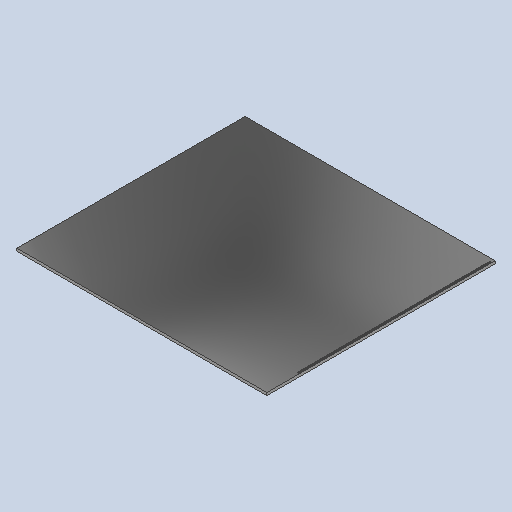
# Autodesk Inventor part: ETROC2
Saved by Autodesk Inventor 2022 (Build 260153000, 153)
## iProperties
Created: 2022-02-01
Part Number: ETROC2
Material: Silicon Nitride
Document SubType Name: Modeling
Designer: Caleb
Density: 3.18 g/cm^3
Appearance: Chrome - Polished Black
Author: Caleb
Autodesk Inventor part; units mm, degrees
ref_plane "YZ Plane" through (0, 0, 0) normal (1, 0, 0) x (0, 1, 0)
ref_plane "XZ Plane" through (0, 0, 0) normal (0, 1, 0) x (-1, 0, 0)
ref_plane "XY Plane" through (0, 0, 0) normal (0, 0, 1) x (1, 0, 0)
sketch "Sketch1" plane through (0, 0, 0) normal (0, 1, 0) x (-1, 0, 0)
  point P0 (0, 0)
sketch "Sketch2" plane through (0, 0, 0) normal (0, 1, 0) x (-1, 0, 0)
  line L0 (-11.5, 10.5) -> (11.5, 10.5)
  line L1 (11.5, 10.5) -> (11.5, -10.5)
  line L2 (11.5, -10.5) -> (-11.5, -10.5)
  line L3 (-11.5, -10.5) -> (-11.5, 10.5)
  line L4 (-11.5, 10.5) -> (11.5, -10.5) construction
  line L5 (11.5, 10.5) -> (-11.5, -10.5) construction
  point P0 (0, 0)
  dimension "d0" = 21
  dimension "d1" = 23
  constraints: 12 end point, 2 midpoint, 2 parallel, 1 horizontal, 1 perpendicular
  measures "d0" distance of L0.end L1.end
  measures "d1" distance of L0.start L0.end
extrude "Extrusion1" add sketch "Sketch2" along normal blind 0.25
sketch "Sketch3" plane through (0, 0.25, 0) normal (0, 1, 0) x (1, 0, 0)
  line L0 (11.5, -10.5) -> (11.5, 10.5) projected
  line L1 (-11.5, -10.5) -> (11.5, -10.5) projected
  line L2 (11.45, -7.5) -> (11.3, -7.5)
  line L3 (11.3, -7.5) -> (11.3, -7.42)
  line L4 (11.3, -7.42) -> (11.45, -7.42)
  line L5 (11.45, -7.42) -> (11.45, -7.5)
  line L6 (11.45, -7.5) -> (11.3, -7.42) construction
  line L7 (11.3, -7.5) -> (11.45, -7.42) construction
  line L8 (11.45, -7.375) -> (11.3, -7.375)
  line L9 (11.3, -7.375) -> (11.3, -7.295)
  line L10 (11.3, -7.295) -> (11.45, -7.295)
  line L11 (11.45, -7.295) -> (11.45, -7.375)
  line L12 (11.45, -7.375) -> (11.3, -7.295) construction
  line L13 (11.3, -7.375) -> (11.45, -7.295) construction
  line L14 (11.45, -7.25) -> (11.3, -7.25)
  line L15 (11.3, -7.25) -> (11.3, -7.17)
  line L16 (11.3, -7.17) -> (11.45, -7.17)
  line L17 (11.45, -7.17) -> (11.45, -7.25)
  line L18 (11.45, -7.25) -> (11.3, -7.17) construction
  line L19 (11.3, -7.25) -> (11.45, -7.17) construction
  line L20 (11.45, -7.125) -> (11.3, -7.125)
  line L21 (11.3, -7.125) -> (11.3, -7.045)
  line L22 (11.3, -7.045) -> (11.45, -7.045)
  line L23 (11.45, -7.045) -> (11.45, -7.125)
  line L24 (11.45, -7.125) -> (11.3, -7.045) construction
  line L25 (11.3, -7.125) -> (11.45, -7.045) construction
  line L26 (11.45, -7) -> (11.3, -7)
  line L27 (11.3, -7) -> (11.3, -6.92)
  line L28 (11.3, -6.92) -> (11.45, -6.92)
  line L29 (11.45, -6.92) -> (11.45, -7)
  line L30 (11.45, -7) -> (11.3, -6.92) construction
  line L31 (11.3, -7) -> (11.45, -6.92) construction
  line L32 (11.45, -6.875) -> (11.3, -6.875)
  line L33 (11.3, -6.875) -> (11.3, -6.795)
  line L34 (11.3, -6.795) -> (11.45, -6.795)
  line L35 (11.45, -6.795) -> (11.45, -6.875)
  line L36 (11.45, -6.875) -> (11.3, -6.795) construction
  line L37 (11.3, -6.875) -> (11.45, -6.795) construction
  line L38 (11.45, -6.75) -> (11.3, -6.75)
  line L39 (11.3, -6.75) -> (11.3, -6.67)
  line L40 (11.3, -6.67) -> (11.45, -6.67)
  line L41 (11.45, -6.67) -> (11.45, -6.75)
  line L42 (11.45, -6.75) -> (11.3, -6.67) construction
  line L43 (11.3, -6.75) -> (11.45, -6.67) construction
  line L44 (11.45, -6.625) -> (11.3, -6.625)
  line L45 (11.3, -6.625) -> (11.3, -6.545)
  line L46 (11.3, -6.545) -> (11.45, -6.545)
  line L47 (11.45, -6.545) -> (11.45, -6.625)
  line L48 (11.45, -6.625) -> (11.3, -6.545) construction
  line L49 (11.3, -6.625) -> (11.45, -6.545) construction
  line L50 (11.45, -6.5) -> (11.3, -6.5)
  line L51 (11.3, -6.5) -> (11.3, -6.42)
  line L52 (11.3, -6.42) -> (11.45, -6.42)
  line L53 (11.45, -6.42) -> (11.45, -6.5)
  line L54 (11.45, -6.5) -> (11.3, -6.42) construction
  line L55 (11.3, -6.5) -> (11.45, -6.42) construction
  line L56 (11.45, -6.375) -> (11.3, -6.375)
  line L57 (11.3, -6.375) -> (11.3, -6.295)
  line L58 (11.3, -6.295) -> (11.45, -6.295)
  line L59 (11.45, -6.295) -> (11.45, -6.375)
  line L60 (11.45, -6.375) -> (11.3, -6.295) construction
  line L61 (11.3, -6.375) -> (11.45, -6.295) construction
  line L62 (11.45, -6.25) -> (11.3, -6.25)
  line L63 (11.3, -6.25) -> (11.3, -6.17)
  line L64 (11.3, -6.17) -> (11.45, -6.17)
  line L65 (11.45, -6.17) -> (11.45, -6.25)
  line L66 (11.45, -6.25) -> (11.3, -6.17) construction
  line L67 (11.3, -6.25) -> (11.45, -6.17) construction
  line L68 (11.45, -6.125) -> (11.3, -6.125)
  line L69 (11.3, -6.125) -> (11.3, -6.045)
  line L70 (11.3, -6.045) -> (11.45, -6.045)
  line L71 (11.45, -6.045) -> (11.45, -6.125)
  line L72 (11.45, -6.125) -> (11.3, -6.045) construction
  line L73 (11.3, -6.125) -> (11.45, -6.045) construction
  line L74 (11.45, -6) -> (11.3, -6)
  line L75 (11.3, -6) -> (11.3, -5.92)
  line L76 (11.3, -5.92) -> (11.45, -5.92)
  line L77 (11.45, -5.92) -> (11.45, -6)
  line L78 (11.45, -6) -> (11.3, -5.92) construction
  line L79 (11.3, -6) -> (11.45, -5.92) construction
  line L80 (11.45, -5.875) -> (11.3, -5.875)
  line L81 (11.3, -5.875) -> (11.3, -5.795)
  line L82 (11.3, -5.795) -> (11.45, -5.795)
  line L83 (11.45, -5.795) -> (11.45, -5.875)
  line L84 (11.45, -5.875) -> (11.3, -5.795) construction
  line L85 (11.3, -5.875) -> (11.45, -5.795) construction
  line L86 (11.45, -5.75) -> (11.3, -5.75)
  line L87 (11.3, -5.75) -> (11.3, -5.67)
  line L88 (11.3, -5.67) -> (11.45, -5.67)
  line L89 (11.45, -5.67) -> (11.45, -5.75)
  line L90 (11.45, -5.75) -> (11.3, -5.67) construction
  line L91 (11.3, -5.75) -> (11.45, -5.67) construction
  line L92 (11.45, -5.625) -> (11.3, -5.625)
  line L93 (11.3, -5.625) -> (11.3, -5.545)
  line L94 (11.3, -5.545) -> (11.45, -5.545)
  line L95 (11.45, -5.545) -> (11.45, -5.625)
  line L96 (11.45, -5.625) -> (11.3, -5.545) construction
  line L97 (11.3, -5.625) -> (11.45, -5.545) construction
  line L98 (11.45, -5.5) -> (11.3, -5.5)
  line L99 (11.3, -5.5) -> (11.3, -5.42)
  line L100 (11.3, -5.42) -> (11.45, -5.42)
  line L101 (11.45, -5.42) -> (11.45, -5.5)
  line L102 (11.45, -5.5) -> (11.3, -5.42) construction
  line L103 (11.3, -5.5) -> (11.45, -5.42) construction
  line L104 (11.45, -5.375) -> (11.3, -5.375)
  line L105 (11.3, -5.375) -> (11.3, -5.295)
  line L106 (11.3, -5.295) -> (11.45, -5.295)
  line L107 (11.45, -5.295) -> (11.45, -5.375)
  line L108 (11.45, -5.375) -> (11.3, -5.295) construction
  line L109 (11.3, -5.375) -> (11.45, -5.295) construction
  line L110 (11.45, -5.25) -> (11.3, -5.25)
  line L111 (11.3, -5.25) -> (11.3, -5.17)
  line L112 (11.3, -5.17) -> (11.45, -5.17)
  line L113 (11.45, -5.17) -> (11.45, -5.25)
  line L114 (11.45, -5.25) -> (11.3, -5.17) construction
  line L115 (11.3, -5.25) -> (11.45, -5.17) construction
  line L116 (11.45, -5.125) -> (11.3, -5.125)
  line L117 (11.3, -5.125) -> (11.3, -5.045)
  line L118 (11.3, -5.045) -> (11.45, -5.045)
  line L119 (11.45, -5.045) -> (11.45, -5.125)
  line L120 (11.45, -5.125) -> (11.3, -5.045) construction
  line L121 (11.3, -5.125) -> (11.45, -5.045) construction
  line L122 (11.45, -5) -> (11.3, -5)
  line L123 (11.3, -5) -> (11.3, -4.92)
  line L124 (11.3, -4.92) -> (11.45, -4.92)
  line L125 (11.45, -4.92) -> (11.45, -5)
  line L126 (11.45, -5) -> (11.3, -4.92) construction
  line L127 (11.3, -5) -> (11.45, -4.92) construction
  line L128 (11.45, -4.875) -> (11.3, -4.875)
  line L129 (11.3, -4.875) -> (11.3, -4.795)
  line L130 (11.3, -4.795) -> (11.45, -4.795)
  line L131 (11.45, -4.795) -> (11.45, -4.875)
  line L132 (11.45, -4.875) -> (11.3, -4.795) construction
  line L133 (11.3, -4.875) -> (11.45, -4.795) construction
  line L134 (11.45, -4.75) -> (11.3, -4.75)
  line L135 (11.3, -4.75) -> (11.3, -4.67)
  line L136 (11.3, -4.67) -> (11.45, -4.67)
  line L137 (11.45, -4.67) -> (11.45, -4.75)
  line L138 (11.45, -4.75) -> (11.3, -4.67) construction
  line L139 (11.3, -4.75) -> (11.45, -4.67) construction
  line L140 (11.45, -4.625) -> (11.3, -4.625)
  line L141 (11.3, -4.625) -> (11.3, -4.545)
  line L142 (11.3, -4.545) -> (11.45, -4.545)
  line L143 (11.45, -4.545) -> (11.45, -4.625)
  line L144 (11.45, -4.625) -> (11.3, -4.545) construction
  line L145 (11.3, -4.625) -> (11.45, -4.545) construction
  line L146 (11.45, -4.5) -> (11.3, -4.5)
  line L147 (11.3, -4.5) -> (11.3, -4.42)
  line L148 (11.3, -4.42) -> (11.45, -4.42)
  line L149 (11.45, -4.42) -> (11.45, -4.5)
  line L150 (11.45, -4.5) -> (11.3, -4.42) construction
  line L151 (11.3, -4.5) -> (11.45, -4.42) construction
  line L152 (11.45, -4.375) -> (11.3, -4.375)
  line L153 (11.3, -4.375) -> (11.3, -4.295)
  line L154 (11.3, -4.295) -> (11.45, -4.295)
  line L155 (11.45, -4.295) -> (11.45, -4.375)
  line L156 (11.45, -4.375) -> (11.3, -4.295) construction
  line L157 (11.3, -4.375) -> (11.45, -4.295) construction
  line L158 (11.45, -4.25) -> (11.3, -4.25)
  line L159 (11.3, -4.25) -> (11.3, -4.17)
  line L160 (11.3, -4.17) -> (11.45, -4.17)
  line L161 (11.45, -4.17) -> (11.45, -4.25)
  line L162 (11.45, -4.25) -> (11.3, -4.17) construction
  line L163 (11.3, -4.25) -> (11.45, -4.17) construction
  line L164 (11.45, -4.125) -> (11.3, -4.125)
  line L165 (11.3, -4.125) -> (11.3, -4.045)
  line L166 (11.3, -4.045) -> (11.45, -4.045)
  line L167 (11.45, -4.045) -> (11.45, -4.125)
  line L168 (11.45, -4.125) -> (11.3, -4.045) construction
  line L169 (11.3, -4.125) -> (11.45, -4.045) construction
  line L170 (11.45, -4) -> (11.3, -4)
  line L171 (11.3, -4) -> (11.3, -3.92)
  line L172 (11.3, -3.92) -> (11.45, -3.92)
  line L173 (11.45, -3.92) -> (11.45, -4)
  line L174 (11.45, -4) -> (11.3, -3.92) construction
  line L175 (11.3, -4) -> (11.45, -3.92) construction
  line L176 (11.45, -3.875) -> (11.3, -3.875)
  line L177 (11.3, -3.875) -> (11.3, -3.795)
  line L178 (11.3, -3.795) -> (11.45, -3.795)
  line L179 (11.45, -3.795) -> (11.45, -3.875)
  line L180 (11.45, -3.875) -> (11.3, -3.795) construction
  line L181 (11.3, -3.875) -> (11.45, -3.795) construction
  line L182 (11.45, -3.75) -> (11.3, -3.75)
  line L183 (11.3, -3.75) -> (11.3, -3.67)
  line L184 (11.3, -3.67) -> (11.45, -3.67)
  line L185 (11.45, -3.67) -> (11.45, -3.75)
  line L186 (11.45, -3.75) -> (11.3, -3.67) construction
  line L187 (11.3, -3.75) -> (11.45, -3.67) construction
  line L188 (11.45, -3.625) -> (11.3, -3.625)
  line L189 (11.3, -3.625) -> (11.3, -3.545)
  line L190 (11.3, -3.545) -> (11.45, -3.545)
  line L191 (11.45, -3.545) -> (11.45, -3.625)
  line L192 (11.45, -3.625) -> (11.3, -3.545) construction
  line L193 (11.3, -3.625) -> (11.45, -3.545) construction
  line L194 (11.45, -3.5) -> (11.3, -3.5)
  line L195 (11.3, -3.5) -> (11.3, -3.42)
  line L196 (11.3, -3.42) -> (11.45, -3.42)
  line L197 (11.45, -3.42) -> (11.45, -3.5)
  line L198 (11.45, -3.5) -> (11.3, -3.42) construction
  line L199 (11.3, -3.5) -> (11.45, -3.42) construction
  line L200 (11.45, -3.375) -> (11.3, -3.375)
  line L201 (11.3, -3.375) -> (11.3, -3.295)
  line L202 (11.3, -3.295) -> (11.45, -3.295)
  line L203 (11.45, -3.295) -> (11.45, -3.375)
  line L204 (11.45, -3.375) -> (11.3, -3.295) construction
  line L205 (11.3, -3.375) -> (11.45, -3.295) construction
  line L206 (11.45, -3.25) -> (11.3, -3.25)
  line L207 (11.3, -3.25) -> (11.3, -3.17)
  line L208 (11.3, -3.17) -> (11.45, -3.17)
  line L209 (11.45, -3.17) -> (11.45, -3.25)
  line L210 (11.45, -3.25) -> (11.3, -3.17) construction
  line L211 (11.3, -3.25) -> (11.45, -3.17) construction
  line L212 (11.45, -3.125) -> (11.3, -3.125)
  line L213 (11.3, -3.125) -> (11.3, -3.045)
  line L214 (11.3, -3.045) -> (11.45, -3.045)
  line L215 (11.45, -3.045) -> (11.45, -3.125)
  line L216 (11.45, -3.125) -> (11.3, -3.045) construction
  line L217 (11.3, -3.125) -> (11.45, -3.045) construction
  line L218 (11.45, -3) -> (11.3, -3)
  line L219 (11.3, -3) -> (11.3, -2.92)
  line L220 (11.3, -2.92) -> (11.45, -2.92)
  line L221 (11.45, -2.92) -> (11.45, -3)
  line L222 (11.45, -3) -> (11.3, -2.92) construction
  line L223 (11.3, -3) -> (11.45, -2.92) construction
  line L224 (11.45, -2.875) -> (11.3, -2.875)
  line L225 (11.3, -2.875) -> (11.3, -2.795)
  line L226 (11.3, -2.795) -> (11.45, -2.795)
  line L227 (11.45, -2.795) -> (11.45, -2.875)
  line L228 (11.45, -2.875) -> (11.3, -2.795) construction
  line L229 (11.3, -2.875) -> (11.45, -2.795) construction
  line L230 (11.45, -2.75) -> (11.3, -2.75)
  line L231 (11.3, -2.75) -> (11.3, -2.67)
  line L232 (11.3, -2.67) -> (11.45, -2.67)
  line L233 (11.45, -2.67) -> (11.45, -2.75)
  line L234 (11.45, -2.75) -> (11.3, -2.67) construction
  line L235 (11.3, -2.75) -> (11.45, -2.67) construction
  line L236 (11.45, -2.625) -> (11.3, -2.625)
  line L237 (11.3, -2.625) -> (11.3, -2.545)
  line L238 (11.3, -2.545) -> (11.45, -2.545)
  line L239 (11.45, -2.545) -> (11.45, -2.625)
  line L240 (11.45, -2.625) -> (11.3, -2.545) construction
  line L241 (11.3, -2.625) -> (11.45, -2.545) construction
  line L242 (11.45, -2.5) -> (11.3, -2.5)
  line L243 (11.3, -2.5) -> (11.3, -2.42)
  line L244 (11.3, -2.42) -> (11.45, -2.42)
  line L245 (11.45, -2.42) -> (11.45, -2.5)
  line L246 (11.45, -2.5) -> (11.3, -2.42) construction
  line L247 (11.3, -2.5) -> (11.45, -2.42) construction
  line L248 (11.45, -2.375) -> (11.3, -2.375)
  line L249 (11.3, -2.375) -> (11.3, -2.295)
  line L250 (11.3, -2.295) -> (11.45, -2.295)
  line L251 (11.45, -2.295) -> (11.45, -2.375)
  line L252 (11.45, -2.375) -> (11.3, -2.295) construction
  line L253 (11.3, -2.375) -> (11.45, -2.295) construction
  line L254 (11.45, -2.25) -> (11.3, -2.25)
  line L255 (11.3, -2.25) -> (11.3, -2.17)
  line L256 (11.3, -2.17) -> (11.45, -2.17)
  line L257 (11.45, -2.17) -> (11.45, -2.25)
  line L258 (11.45, -2.25) -> (11.3, -2.17) construction
  line L259 (11.3, -2.25) -> (11.45, -2.17) construction
  line L260 (11.45, -2.125) -> (11.3, -2.125)
  line L261 (11.3, -2.125) -> (11.3, -2.045)
  line L262 (11.3, -2.045) -> (11.45, -2.045)
  line L263 (11.45, -2.045) -> (11.45, -2.125)
  line L264 (11.45, -2.125) -> (11.3, -2.045) construction
  line L265 (11.3, -2.125) -> (11.45, -2.045) construction
  line L266 (11.45, -2) -> (11.3, -2)
  line L267 (11.3, -2) -> (11.3, -1.92)
  line L268 (11.3, -1.92) -> (11.45, -1.92)
  line L269 (11.45, -1.92) -> (11.45, -2)
  line L270 (11.45, -2) -> (11.3, -1.92) construction
  line L271 (11.3, -2) -> (11.45, -1.92) construction
  line L272 (11.45, -1.875) -> (11.3, -1.875)
  line L273 (11.3, -1.875) -> (11.3, -1.795)
  line L274 (11.3, -1.795) -> (11.45, -1.795)
  line L275 (11.45, -1.795) -> (11.45, -1.875)
  line L276 (11.45, -1.875) -> (11.3, -1.795) construction
  line L277 (11.3, -1.875) -> (11.45, -1.795) construction
  line L278 (11.45, -1.75) -> (11.3, -1.75)
  line L279 (11.3, -1.75) -> (11.3, -1.67)
  line L280 (11.3, -1.67) -> (11.45, -1.67)
  line L281 (11.45, -1.67) -> (11.45, -1.75)
  line L282 (11.45, -1.75) -> (11.3, -1.67) construction
  line L283 (11.3, -1.75) -> (11.45, -1.67) construction
  line L284 (11.45, -1.625) -> (11.3, -1.625)
  line L285 (11.3, -1.625) -> (11.3, -1.545)
  line L286 (11.3, -1.545) -> (11.45, -1.545)
  line L287 (11.45, -1.545) -> (11.45, -1.625)
  line L288 (11.45, -1.625) -> (11.3, -1.545) construction
  line L289 (11.3, -1.625) -> (11.45, -1.545) construction
  line L290 (11.45, -1.5) -> (11.3, -1.5)
  line L291 (11.3, -1.5) -> (11.3, -1.42)
  line L292 (11.3, -1.42) -> (11.45, -1.42)
  line L293 (11.45, -1.42) -> (11.45, -1.5)
  line L294 (11.45, -1.5) -> (11.3, -1.42) construction
  line L295 (11.3, -1.5) -> (11.45, -1.42) construction
  line L296 (11.45, -1.375) -> (11.3, -1.375)
  line L297 (11.3, -1.375) -> (11.3, -1.295)
  line L298 (11.3, -1.295) -> (11.45, -1.295)
  line L299 (11.45, -1.295) -> (11.45, -1.375)
  line L300 (11.45, -1.375) -> (11.3, -1.295) construction
  line L301 (11.3, -1.375) -> (11.45, -1.295) construction
  line L302 (11.45, -1.25) -> (11.3, -1.25)
  line L303 (11.3, -1.25) -> (11.3, -1.17)
  line L304 (11.3, -1.17) -> (11.45, -1.17)
  line L305 (11.45, -1.17) -> (11.45, -1.25)
  line L306 (11.45, -1.25) -> (11.3, -1.17) construction
  line L307 (11.3, -1.25) -> (11.45, -1.17) construction
  line L308 (11.45, -1.125) -> (11.3, -1.125)
  line L309 (11.3, -1.125) -> (11.3, -1.045)
  line L310 (11.3, -1.045) -> (11.45, -1.045)
  line L311 (11.45, -1.045) -> (11.45, -1.125)
  line L312 (11.45, -1.125) -> (11.3, -1.045) construction
  line L313 (11.3, -1.125) -> (11.45, -1.045) construction
  line L314 (11.45, -1) -> (11.3, -1)
  line L315 (11.3, -1) -> (11.3, -0.92)
  line L316 (11.3, -0.92) -> (11.45, -0.92)
  line L317 (11.45, -0.92) -> (11.45, -1)
  line L318 (11.45, -1) -> (11.3, -0.92) construction
  line L319 (11.3, -1) -> (11.45, -0.92) construction
  line L320 (11.45, -0.875) -> (11.3, -0.875)
  line L321 (11.3, -0.875) -> (11.3, -0.795)
  line L322 (11.3, -0.795) -> (11.45, -0.795)
  line L323 (11.45, -0.795) -> (11.45, -0.875)
  line L324 (11.45, -0.875) -> (11.3, -0.795) construction
  line L325 (11.3, -0.875) -> (11.45, -0.795) construction
  line L326 (11.45, -0.75) -> (11.3, -0.75)
  line L327 (11.3, -0.75) -> (11.3, -0.67)
  line L328 (11.3, -0.67) -> (11.45, -0.67)
  line L329 (11.45, -0.67) -> (11.45, -0.75)
  line L330 (11.45, -0.75) -> (11.3, -0.67) construction
  line L331 (11.3, -0.75) -> (11.45, -0.67) construction
  line L332 (11.45, -0.625) -> (11.3, -0.625)
  line L333 (11.3, -0.625) -> (11.3, -0.545)
  line L334 (11.3, -0.545) -> (11.45, -0.545)
  line L335 (11.45, -0.545) -> (11.45, -0.625)
  line L336 (11.45, -0.625) -> (11.3, -0.545) construction
  line L337 (11.3, -0.625) -> (11.45, -0.545) construction
  line L338 (11.45, -0.5) -> (11.3, -0.5)
  line L339 (11.3, -0.5) -> (11.3, -0.42)
  line L340 (11.3, -0.42) -> (11.45, -0.42)
  line L341 (11.45, -0.42) -> (11.45, -0.5)
  line L342 (11.45, -0.5) -> (11.3, -0.42) construction
  line L343 (11.3, -0.5) -> (11.45, -0.42) construction
  line L344 (11.45, -0.375) -> (11.3, -0.375)
  line L345 (11.3, -0.375) -> (11.3, -0.295)
  line L346 (11.3, -0.295) -> (11.45, -0.295)
  line L347 (11.45, -0.295) -> (11.45, -0.375)
  line L348 (11.45, -0.375) -> (11.3, -0.295) construction
  line L349 (11.3, -0.375) -> (11.45, -0.295) construction
  line L350 (11.45, -0.25) -> (11.3, -0.25)
  line L351 (11.3, -0.25) -> (11.3, -0.17)
  line L352 (11.3, -0.17) -> (11.45, -0.17)
  line L353 (11.45, -0.17) -> (11.45, -0.25)
  line L354 (11.45, -0.25) -> (11.3, -0.17) construction
  line L355 (11.3, -0.25) -> (11.45, -0.17) construction
  line L356 (11.45, -0.125) -> (11.3, -0.125)
  line L357 (11.3, -0.125) -> (11.3, -0.045)
  line L358 (11.3, -0.045) -> (11.45, -0.045)
  line L359 (11.45, -0.045) -> (11.45, -0.125)
  line L360 (11.45, -0.125) -> (11.3, -0.045) construction
  line L361 (11.3, -0.125) -> (11.45, -0.045) construction
  line L362 (11.45, 0) -> (11.3, 0)
  line L363 (11.3, 0) -> (11.3, 0.08)
  line L364 (11.3, 0.08) -> (11.45, 0.08)
  line L365 (11.45, 0.08) -> (11.45, 0)
  line L366 (11.45, 0) -> (11.3, 0.08) construction
  line L367 (11.3, 0) -> (11.45, 0.08) construction
  line L368 (11.45, 0.125) -> (11.3, 0.125)
  line L369 (11.3, 0.125) -> (11.3, 0.205)
  line L370 (11.3, 0.205) -> (11.45, 0.205)
  line L371 (11.45, 0.205) -> (11.45, 0.125)
  line L372 (11.45, 0.125) -> (11.3, 0.205) construction
  line L373 (11.3, 0.125) -> (11.45, 0.205) construction
  line L374 (11.45, 0.25) -> (11.3, 0.25)
  line L375 (11.3, 0.25) -> (11.3, 0.33)
  line L376 (11.3, 0.33) -> (11.45, 0.33)
  line L377 (11.45, 0.33) -> (11.45, 0.25)
  line L378 (11.45, 0.25) -> (11.3, 0.33) construction
  line L379 (11.3, 0.25) -> (11.45, 0.33) construction
  line L380 (11.45, 0.375) -> (11.3, 0.375)
  line L381 (11.3, 0.375) -> (11.3, 0.455)
  line L382 (11.3, 0.455) -> (11.45, 0.455)
  line L383 (11.45, 0.455) -> (11.45, 0.375)
  line L384 (11.45, 0.375) -> (11.3, 0.455) construction
  line L385 (11.3, 0.375) -> (11.45, 0.455) construction
  line L386 (11.45, 0.5) -> (11.3, 0.5)
  line L387 (11.3, 0.5) -> (11.3, 0.58)
  line L388 (11.3, 0.58) -> (11.45, 0.58)
  line L389 (11.45, 0.58) -> (11.45, 0.5)
  line L390 (11.45, 0.5) -> (11.3, 0.58) construction
  line L391 (11.3, 0.5) -> (11.45, 0.58) construction
  line L392 (11.45, 0.625) -> (11.3, 0.625)
  line L393 (11.3, 0.625) -> (11.3, 0.705)
  line L394 (11.3, 0.705) -> (11.45, 0.705)
  line L395 (11.45, 0.705) -> (11.45, 0.625)
  line L396 (11.45, 0.625) -> (11.3, 0.705) construction
  line L397 (11.3, 0.625) -> (11.45, 0.705) construction
  line L398 (11.45, 0.75) -> (11.3, 0.75)
  line L399 (11.3, 0.75) -> (11.3, 0.83)
  line L400 (11.3, 0.83) -> (11.45, 0.83)
  line L401 (11.45, 0.83) -> (11.45, 0.75)
  line L402 (11.45, 0.75) -> (11.3, 0.83) construction
  line L403 (11.3, 0.75) -> (11.45, 0.83) construction
  line L404 (11.45, 0.875) -> (11.3, 0.875)
  line L405 (11.3, 0.875) -> (11.3, 0.955)
  line L406 (11.3, 0.955) -> (11.45, 0.955)
  line L407 (11.45, 0.955) -> (11.45, 0.875)
  line L408 (11.45, 0.875) -> (11.3, 0.955) construction
  line L409 (11.3, 0.875) -> (11.45, 0.955) construction
  line L410 (11.45, 1) -> (11.3, 1)
  line L411 (11.3, 1) -> (11.3, 1.08)
  line L412 (11.3, 1.08) -> (11.45, 1.08)
  line L413 (11.45, 1.08) -> (11.45, 1)
  line L414 (11.45, 1) -> (11.3, 1.08) construction
  line L415 (11.3, 1) -> (11.45, 1.08) construction
  line L416 (11.45, 1.125) -> (11.3, 1.125)
  line L417 (11.3, 1.125) -> (11.3, 1.205)
  line L418 (11.3, 1.205) -> (11.45, 1.205)
  line L419 (11.45, 1.205) -> (11.45, 1.125)
  line L420 (11.45, 1.125) -> (11.3, 1.205) construction
  line L421 (11.3, 1.125) -> (11.45, 1.205) construction
  line L422 (11.45, 1.25) -> (11.3, 1.25)
  line L423 (11.3, 1.25) -> (11.3, 1.33)
  line L424 (11.3, 1.33) -> (11.45, 1.33)
  line L425 (11.45, 1.33) -> (11.45, 1.25)
  line L426 (11.45, 1.25) -> (11.3, 1.33) construction
  line L427 (11.3, 1.25) -> (11.45, 1.33) construction
  line L428 (11.45, 1.375) -> (11.3, 1.375)
  line L429 (11.3, 1.375) -> (11.3, 1.455)
  line L430 (11.3, 1.455) -> (11.45, 1.455)
  line L431 (11.45, 1.455) -> (11.45, 1.375)
  line L432 (11.45, 1.375) -> (11.3, 1.455) construction
  line L433 (11.3, 1.375) -> (11.45, 1.455) construction
  line L434 (11.45, 1.5) -> (11.3, 1.5)
  line L435 (11.3, 1.5) -> (11.3, 1.58)
  line L436 (11.3, 1.58) -> (11.45, 1.58)
  line L437 (11.45, 1.58) -> (11.45, 1.5)
  line L438 (11.45, 1.5) -> (11.3, 1.58) construction
  line L439 (11.3, 1.5) -> (11.45, 1.58) construction
  line L440 (11.45, 1.625) -> (11.3, 1.625)
  line L441 (11.3, 1.625) -> (11.3, 1.705)
  line L442 (11.3, 1.705) -> (11.45, 1.705)
  line L443 (11.45, 1.705) -> (11.45, 1.625)
  line L444 (11.45, 1.625) -> (11.3, 1.705) construction
  line L445 (11.3, 1.625) -> (11.45, 1.705) construction
  line L446 (11.45, 1.75) -> (11.3, 1.75)
  line L447 (11.3, 1.75) -> (11.3, 1.83)
  line L448 (11.3, 1.83) -> (11.45, 1.83)
  line L449 (11.45, 1.83) -> (11.45, 1.75)
  line L450 (11.45, 1.75) -> (11.3, 1.83) construction
  line L451 (11.3, 1.75) -> (11.45, 1.83) construction
  line L452 (11.45, 1.875) -> (11.3, 1.875)
  line L453 (11.3, 1.875) -> (11.3, 1.955)
  line L454 (11.3, 1.955) -> (11.45, 1.955)
  line L455 (11.45, 1.955) -> (11.45, 1.875)
  line L456 (11.45, 1.875) -> (11.3, 1.955) construction
  line L457 (11.3, 1.875) -> (11.45, 1.955) construction
  line L458 (11.45, 2) -> (11.3, 2)
  line L459 (11.3, 2) -> (11.3, 2.08)
  line L460 (11.3, 2.08) -> (11.45, 2.08)
  line L461 (11.45, 2.08) -> (11.45, 2)
  line L462 (11.45, 2) -> (11.3, 2.08) construction
  line L463 (11.3, 2) -> (11.45, 2.08) construction
  line L464 (11.45, 2.125) -> (11.3, 2.125)
  line L465 (11.3, 2.125) -> (11.3, 2.205)
  line L466 (11.3, 2.205) -> (11.45, 2.205)
  line L467 (11.45, 2.205) -> (11.45, 2.125)
  line L468 (11.45, 2.125) -> (11.3, 2.205) construction
  line L469 (11.3, 2.125) -> (11.45, 2.205) construction
  line L470 (11.45, 2.25) -> (11.3, 2.25)
  line L471 (11.3, 2.25) -> (11.3, 2.33)
  line L472 (11.3, 2.33) -> (11.45, 2.33)
  line L473 (11.45, 2.33) -> (11.45, 2.25)
  line L474 (11.45, 2.25) -> (11.3, 2.33) construction
  line L475 (11.3, 2.25) -> (11.45, 2.33) construction
  line L476 (11.45, 2.375) -> (11.3, 2.375)
  line L477 (11.3, 2.375) -> (11.3, 2.455)
  line L478 (11.3, 2.455) -> (11.45, 2.455)
  line L479 (11.45, 2.455) -> (11.45, 2.375)
  line L480 (11.45, 2.375) -> (11.3, 2.455) construction
  line L481 (11.3, 2.375) -> (11.45, 2.455) construction
  line L482 (11.45, 2.5) -> (11.3, 2.5)
  line L483 (11.3, 2.5) -> (11.3, 2.58)
  line L484 (11.3, 2.58) -> (11.45, 2.58)
  line L485 (11.45, 2.58) -> (11.45, 2.5)
  line L486 (11.45, 2.5) -> (11.3, 2.58) construction
  line L487 (11.3, 2.5) -> (11.45, 2.58) construction
  line L488 (11.45, 2.625) -> (11.3, 2.625)
  line L489 (11.3, 2.625) -> (11.3, 2.705)
  line L490 (11.3, 2.705) -> (11.45, 2.705)
  line L491 (11.45, 2.705) -> (11.45, 2.625)
  line L492 (11.45, 2.625) -> (11.3, 2.705) construction
  line L493 (11.3, 2.625) -> (11.45, 2.705) construction
  line L494 (11.45, 2.75) -> (11.3, 2.75)
  line L495 (11.3, 2.75) -> (11.3, 2.83)
  line L496 (11.3, 2.83) -> (11.45, 2.83)
  line L497 (11.45, 2.83) -> (11.45, 2.75)
  line L498 (11.45, 2.75) -> (11.3, 2.83) construction
  line L499 (11.3, 2.75) -> (11.45, 2.83) construction
  line L500 (11.45, 2.875) -> (11.3, 2.875)
  line L501 (11.3, 2.875) -> (11.3, 2.955)
  line L502 (11.3, 2.955) -> (11.45, 2.955)
  line L503 (11.45, 2.955) -> (11.45, 2.875)
  line L504 (11.45, 2.875) -> (11.3, 2.955) construction
  line L505 (11.3, 2.875) -> (11.45, 2.955) construction
  line L506 (11.45, 3) -> (11.3, 3)
  line L507 (11.3, 3) -> (11.3, 3.08)
  line L508 (11.3, 3.08) -> (11.45, 3.08)
  line L509 (11.45, 3.08) -> (11.45, 3)
  line L510 (11.45, 3) -> (11.3, 3.08) construction
  line L511 (11.3, 3) -> (11.45, 3.08) construction
  line L512 (11.45, 3.125) -> (11.3, 3.125)
  line L513 (11.3, 3.125) -> (11.3, 3.205)
  line L514 (11.3, 3.205) -> (11.45, 3.205)
  line L515 (11.45, 3.205) -> (11.45, 3.125)
  line L516 (11.45, 3.125) -> (11.3, 3.205) construction
  line L517 (11.3, 3.125) -> (11.45, 3.205) construction
  line L518 (11.45, 3.25) -> (11.3, 3.25)
  line L519 (11.3, 3.25) -> (11.3, 3.33)
  line L520 (11.3, 3.33) -> (11.45, 3.33)
  line L521 (11.45, 3.33) -> (11.45, 3.25)
  line L522 (11.45, 3.25) -> (11.3, 3.33) construction
  line L523 (11.3, 3.25) -> (11.45, 3.33) construction
  line L524 (11.45, 3.375) -> (11.3, 3.375)
  line L525 (11.3, 3.375) -> (11.3, 3.455)
  line L526 (11.3, 3.455) -> (11.45, 3.455)
  line L527 (11.45, 3.455) -> (11.45, 3.375)
  line L528 (11.45, 3.375) -> (11.3, 3.455) construction
  line L529 (11.3, 3.375) -> (11.45, 3.455) construction
  line L530 (11.45, 3.5) -> (11.3, 3.5)
  line L531 (11.3, 3.5) -> (11.3, 3.58)
  line L532 (11.3, 3.58) -> (11.45, 3.58)
  line L533 (11.45, 3.58) -> (11.45, 3.5)
  line L534 (11.45, 3.5) -> (11.3, 3.58) construction
  line L535 (11.3, 3.5) -> (11.45, 3.58) construction
  line L536 (11.45, 3.625) -> (11.3, 3.625)
  line L537 (11.3, 3.625) -> (11.3, 3.705)
  line L538 (11.3, 3.705) -> (11.45, 3.705)
  line L539 (11.45, 3.705) -> (11.45, 3.625)
  line L540 (11.45, 3.625) -> (11.3, 3.705) construction
  line L541 (11.3, 3.625) -> (11.45, 3.705) construction
  line L542 (11.45, 3.75) -> (11.3, 3.75)
  line L543 (11.3, 3.75) -> (11.3, 3.83)
  line L544 (11.3, 3.83) -> (11.45, 3.83)
  line L545 (11.45, 3.83) -> (11.45, 3.75)
  line L546 (11.45, 3.75) -> (11.3, 3.83) construction
  line L547 (11.3, 3.75) -> (11.45, 3.83) construction
  line L548 (11.45, 3.875) -> (11.3, 3.875)
  line L549 (11.3, 3.875) -> (11.3, 3.955)
  line L550 (11.3, 3.955) -> (11.45, 3.955)
  line L551 (11.45, 3.955) -> (11.45, 3.875)
  line L552 (11.45, 3.875) -> (11.3, 3.955) construction
  line L553 (11.3, 3.875) -> (11.45, 3.955) construction
  line L554 (11.45, 4) -> (11.3, 4)
  line L555 (11.3, 4) -> (11.3, 4.08)
  line L556 (11.3, 4.08) -> (11.45, 4.08)
  line L557 (11.45, 4.08) -> (11.45, 4)
  line L558 (11.45, 4) -> (11.3, 4.08) construction
  line L559 (11.3, 4) -> (11.45, 4.08) construction
  line L560 (11.45, 4.125) -> (11.3, 4.125)
  line L561 (11.3, 4.125) -> (11.3, 4.205)
  line L562 (11.3, 4.205) -> (11.45, 4.205)
  line L563 (11.45, 4.205) -> (11.45, 4.125)
  line L564 (11.45, 4.125) -> (11.3, 4.205) construction
  line L565 (11.3, 4.125) -> (11.45, 4.205) construction
  line L566 (11.45, 4.25) -> (11.3, 4.25)
  line L567 (11.3, 4.25) -> (11.3, 4.33)
  line L568 (11.3, 4.33) -> (11.45, 4.33)
  line L569 (11.45, 4.33) -> (11.45, 4.25)
  line L570 (11.45, 4.25) -> (11.3, 4.33) construction
  line L571 (11.3, 4.25) -> (11.45, 4.33) construction
  line L572 (11.45, 4.375) -> (11.3, 4.375)
  line L573 (11.3, 4.375) -> (11.3, 4.455)
  line L574 (11.3, 4.455) -> (11.45, 4.455)
  line L575 (11.45, 4.455) -> (11.45, 4.375)
  line L576 (11.45, 4.375) -> (11.3, 4.455) construction
  line L577 (11.3, 4.375) -> (11.45, 4.455) construction
  line L578 (11.45, 4.5) -> (11.3, 4.5)
  line L579 (11.3, 4.5) -> (11.3, 4.58)
  line L580 (11.3, 4.58) -> (11.45, 4.58)
  line L581 (11.45, 4.58) -> (11.45, 4.5)
  line L582 (11.45, 4.5) -> (11.3, 4.58) construction
  line L583 (11.3, 4.5) -> (11.45, 4.58) construction
  line L584 (11.45, 4.625) -> (11.3, 4.625)
  line L585 (11.3, 4.625) -> (11.3, 4.705)
  line L586 (11.3, 4.705) -> (11.45, 4.705)
  line L587 (11.45, 4.705) -> (11.45, 4.625)
  line L588 (11.45, 4.625) -> (11.3, 4.705) construction
  line L589 (11.3, 4.625) -> (11.45, 4.705) construction
  line L590 (11.45, 4.75) -> (11.3, 4.75)
  line L591 (11.3, 4.75) -> (11.3, 4.83)
  line L592 (11.3, 4.83) -> (11.45, 4.83)
  line L593 (11.45, 4.83) -> (11.45, 4.75)
  line L594 (11.45, 4.75) -> (11.3, 4.83) construction
  line L595 (11.3, 4.75) -> (11.45, 4.83) construction
  line L596 (11.45, 4.875) -> (11.3, 4.875)
  line L597 (11.3, 4.875) -> (11.3, 4.955)
  line L598 (11.3, 4.955) -> (11.45, 4.955)
  line L599 (11.45, 4.955) -> (11.45, 4.875)
  line L600 (11.45, 4.875) -> (11.3, 4.955) construction
  line L601 (11.3, 4.875) -> (11.45, 4.955) construction
  line L602 (11.45, 5) -> (11.3, 5)
  line L603 (11.3, 5) -> (11.3, 5.08)
  line L604 (11.3, 5.08) -> (11.45, 5.08)
  line L605 (11.45, 5.08) -> (11.45, 5)
  line L606 (11.45, 5) -> (11.3, 5.08) construction
  line L607 (11.3, 5) -> (11.45, 5.08) construction
  line L608 (11.45, 5.125) -> (11.3, 5.125)
  line L609 (11.3, 5.125) -> (11.3, 5.205)
  line L610 (11.3, 5.205) -> (11.45, 5.205)
  line L611 (11.45, 5.205) -> (11.45, 5.125)
  line L612 (11.45, 5.125) -> (11.3, 5.205) construction
  line L613 (11.3, 5.125) -> (11.45, 5.205) construction
  line L614 (11.45, 5.25) -> (11.3, 5.25)
  line L615 (11.3, 5.25) -> (11.3, 5.33)
  line L616 (11.3, 5.33) -> (11.45, 5.33)
  line L617 (11.45, 5.33) -> (11.45, 5.25)
  line L618 (11.45, 5.25) -> (11.3, 5.33) construction
  line L619 (11.3, 5.25) -> (11.45, 5.33) construction
  line L620 (11.45, 5.375) -> (11.3, 5.375)
  line L621 (11.3, 5.375) -> (11.3, 5.455)
  line L622 (11.3, 5.455) -> (11.45, 5.455)
  line L623 (11.45, 5.455) -> (11.45, 5.375)
  line L624 (11.45, 5.375) -> (11.3, 5.455) construction
  line L625 (11.3, 5.375) -> (11.45, 5.455) construction
  line L626 (11.45, 5.5) -> (11.3, 5.5)
  line L627 (11.3, 5.5) -> (11.3, 5.58)
  line L628 (11.3, 5.58) -> (11.45, 5.58)
  line L629 (11.45, 5.58) -> (11.45, 5.5)
  line L630 (11.45, 5.5) -> (11.3, 5.58) construction
  line L631 (11.3, 5.5) -> (11.45, 5.58) construction
  line L632 (11.45, 5.625) -> (11.3, 5.625)
  line L633 (11.3, 5.625) -> (11.3, 5.705)
  line L634 (11.3, 5.705) -> (11.45, 5.705)
  line L635 (11.45, 5.705) -> (11.45, 5.625)
  line L636 (11.45, 5.625) -> (11.3, 5.705) construction
  line L637 (11.3, 5.625) -> (11.45, 5.705) construction
  line L638 (11.45, 5.75) -> (11.3, 5.75)
  line L639 (11.3, 5.75) -> (11.3, 5.83)
  line L640 (11.3, 5.83) -> (11.45, 5.83)
  line L641 (11.45, 5.83) -> (11.45, 5.75)
  line L642 (11.45, 5.75) -> (11.3, 5.83) construction
  line L643 (11.3, 5.75) -> (11.45, 5.83) construction
  line L644 (11.45, 5.875) -> (11.3, 5.875)
  line L645 (11.3, 5.875) -> (11.3, 5.955)
  line L646 (11.3, 5.955) -> (11.45, 5.955)
  line L647 (11.45, 5.955) -> (11.45, 5.875)
  line L648 (11.45, 5.875) -> (11.3, 5.955) construction
  line L649 (11.3, 5.875) -> (11.45, 5.955) construction
  line L650 (11.45, 6) -> (11.3, 6)
  line L651 (11.3, 6) -> (11.3, 6.08)
  line L652 (11.3, 6.08) -> (11.45, 6.08)
  line L653 (11.45, 6.08) -> (11.45, 6)
  line L654 (11.45, 6) -> (11.3, 6.08) construction
  line L655 (11.3, 6) -> (11.45, 6.08) construction
  line L656 (11.45, 6.125) -> (11.3, 6.125)
  line L657 (11.3, 6.125) -> (11.3, 6.205)
  line L658 (11.3, 6.205) -> (11.45, 6.205)
  line L659 (11.45, 6.205) -> (11.45, 6.125)
  line L660 (11.45, 6.125) -> (11.3, 6.205) construction
  line L661 (11.3, 6.125) -> (11.45, 6.205) construction
  line L662 (11.45, 6.25) -> (11.3, 6.25)
  line L663 (11.3, 6.25) -> (11.3, 6.33)
  line L664 (11.3, 6.33) -> (11.45, 6.33)
  line L665 (11.45, 6.33) -> (11.45, 6.25)
  line L666 (11.45, 6.25) -> (11.3, 6.33) construction
  line L667 (11.3, 6.25) -> (11.45, 6.33) construction
  line L668 (11.45, 6.375) -> (11.3, 6.375)
  line L669 (11.3, 6.375) -> (11.3, 6.455)
  line L670 (11.3, 6.455) -> (11.45, 6.455)
  line L671 (11.45, 6.455) -> (11.45, 6.375)
  line L672 (11.45, 6.375) -> (11.3, 6.455) construction
  line L673 (11.3, 6.375) -> (11.45, 6.455) construction
  line L674 (11.45, 6.5) -> (11.3, 6.5)
  line L675 (11.3, 6.5) -> (11.3, 6.58)
  line L676 (11.3, 6.58) -> (11.45, 6.58)
  line L677 (11.45, 6.58) -> (11.45, 6.5)
  line L678 (11.45, 6.5) -> (11.3, 6.58) construction
  line L679 (11.3, 6.5) -> (11.45, 6.58) construction
  line L680 (11.45, 6.625) -> (11.3, 6.625)
  line L681 (11.3, 6.625) -> (11.3, 6.705)
  line L682 (11.3, 6.705) -> (11.45, 6.705)
  line L683 (11.45, 6.705) -> (11.45, 6.625)
  line L684 (11.45, 6.625) -> (11.3, 6.705) construction
  line L685 (11.3, 6.625) -> (11.45, 6.705) construction
  line L686 (11.45, 6.75) -> (11.3, 6.75)
  line L687 (11.3, 6.75) -> (11.3, 6.83)
  line L688 (11.3, 6.83) -> (11.45, 6.83)
  line L689 (11.45, 6.83) -> (11.45, 6.75)
  line L690 (11.45, 6.75) -> (11.3, 6.83) construction
  line L691 (11.3, 6.75) -> (11.45, 6.83) construction
  line L692 (11.45, 6.875) -> (11.3, 6.875)
  line L693 (11.3, 6.875) -> (11.3, 6.955)
  line L694 (11.3, 6.955) -> (11.45, 6.955)
  line L695 (11.45, 6.955) -> (11.45, 6.875)
  line L696 (11.45, 6.875) -> (11.3, 6.955) construction
  line L697 (11.3, 6.875) -> (11.45, 6.955) construction
  line L698 (11.45, 7) -> (11.3, 7)
  line L699 (11.3, 7) -> (11.3, 7.08)
  line L700 (11.3, 7.08) -> (11.45, 7.08)
  line L701 (11.45, 7.08) -> (11.45, 7)
  line L702 (11.45, 7) -> (11.3, 7.08) construction
  line L703 (11.3, 7) -> (11.45, 7.08) construction
  line L704 (11.45, 7.125) -> (11.3, 7.125)
  line L705 (11.3, 7.125) -> (11.3, 7.205)
  line L706 (11.3, 7.205) -> (11.45, 7.205)
  line L707 (11.45, 7.205) -> (11.45, 7.125)
  line L708 (11.45, 7.125) -> (11.3, 7.205) construction
  line L709 (11.3, 7.125) -> (11.45, 7.205) construction
  line L710 (11.45, 7.25) -> (11.3, 7.25)
  line L711 (11.3, 7.25) -> (11.3, 7.33)
  line L712 (11.3, 7.33) -> (11.45, 7.33)
  line L713 (11.45, 7.33) -> (11.45, 7.25)
  line L714 (11.45, 7.25) -> (11.3, 7.33) construction
  line L715 (11.3, 7.25) -> (11.45, 7.33) construction
  line L716 (11.45, 7.375) -> (11.3, 7.375)
  line L717 (11.3, 7.375) -> (11.3, 7.455)
  line L718 (11.3, 7.455) -> (11.45, 7.455)
  line L719 (11.45, 7.455) -> (11.45, 7.375)
  line L720 (11.45, 7.375) -> (11.3, 7.455) construction
  line L721 (11.3, 7.375) -> (11.45, 7.455) construction
  line L722 (11.45, 7.5) -> (11.3, 7.5)
  line L723 (11.3, 7.5) -> (11.3, 7.58)
  line L724 (11.3, 7.58) -> (11.45, 7.58)
  line L725 (11.45, 7.58) -> (11.45, 7.5)
  line L726 (11.45, 7.5) -> (11.3, 7.58) construction
  line L727 (11.3, 7.5) -> (11.45, 7.58) construction
  line L728 (11.45, 7.625) -> (11.3, 7.625)
  line L729 (11.3, 7.625) -> (11.3, 7.705)
  line L730 (11.3, 7.705) -> (11.45, 7.705)
  line L731 (11.45, 7.705) -> (11.45, 7.625)
  line L732 (11.45, 7.625) -> (11.3, 7.705) construction
  line L733 (11.3, 7.625) -> (11.45, 7.705) construction
  line L734 (11.45, 7.75) -> (11.3, 7.75)
  line L735 (11.3, 7.75) -> (11.3, 7.83)
  line L736 (11.3, 7.83) -> (11.45, 7.83)
  line L737 (11.45, 7.83) -> (11.45, 7.75)
  line L738 (11.45, 7.75) -> (11.3, 7.83) construction
  line L739 (11.3, 7.75) -> (11.45, 7.83) construction
  line L740 (11.45, 7.875) -> (11.3, 7.875)
  line L741 (11.3, 7.875) -> (11.3, 7.955)
  line L742 (11.3, 7.955) -> (11.45, 7.955)
  line L743 (11.45, 7.955) -> (11.45, 7.875)
  line L744 (11.45, 7.875) -> (11.3, 7.955) construction
  line L745 (11.3, 7.875) -> (11.45, 7.955) construction
  line L746 (11.45, 8) -> (11.3, 8)
  line L747 (11.3, 8) -> (11.3, 8.08)
  line L748 (11.3, 8.08) -> (11.45, 8.08)
  line L749 (11.45, 8.08) -> (11.45, 8)
  line L750 (11.45, 8) -> (11.3, 8.08) construction
  line L751 (11.3, 8) -> (11.45, 8.08) construction
  line L752 (11.45, 8.125) -> (11.3, 8.125)
  line L753 (11.3, 8.125) -> (11.3, 8.205)
  line L754 (11.3, 8.205) -> (11.45, 8.205)
  line L755 (11.45, 8.205) -> (11.45, 8.125)
  line L756 (11.45, 8.125) -> (11.3, 8.205) construction
  line L757 (11.3, 8.125) -> (11.45, 8.205) construction
  line L758 (11.45, 8.25) -> (11.3, 8.25)
  line L759 (11.3, 8.25) -> (11.3, 8.33)
  line L760 (11.3, 8.33) -> (11.45, 8.33)
  line L761 (11.45, 8.33) -> (11.45, 8.25)
  line L762 (11.45, 8.25) -> (11.3, 8.33) construction
  line L763 (11.3, 8.25) -> (11.45, 8.33) construction
  line L764 (11.45, 8.375) -> (11.3, 8.375)
  line L765 (11.3, 8.375) -> (11.3, 8.455)
  line L766 (11.3, 8.455) -> (11.45, 8.455)
  line L767 (11.45, 8.455) -> (11.45, 8.375)
  line L768 (11.45, 8.375) -> (11.3, 8.455) construction
  line L769 (11.3, 8.375) -> (11.45, 8.455) construction
  line L770 (11.45, 8.5) -> (11.3, 8.5)
  line L771 (11.3, 8.5) -> (11.3, 8.58)
  line L772 (11.3, 8.58) -> (11.45, 8.58)
  line L773 (11.45, 8.58) -> (11.45, 8.5)
  line L774 (11.45, 8.5) -> (11.3, 8.58) construction
  line L775 (11.3, 8.5) -> (11.45, 8.58) construction
  line L776 (11.45, 8.625) -> (11.3, 8.625)
  line L777 (11.3, 8.625) -> (11.3, 8.705)
  line L778 (11.3, 8.705) -> (11.45, 8.705)
  line L779 (11.45, 8.705) -> (11.45, 8.625)
  line L780 (11.45, 8.625) -> (11.3, 8.705) construction
  line L781 (11.3, 8.625) -> (11.45, 8.705) construction
  line L782 (11.45, 8.75) -> (11.3, 8.75)
  line L783 (11.3, 8.75) -> (11.3, 8.83)
  line L784 (11.3, 8.83) -> (11.45, 8.83)
  line L785 (11.45, 8.83) -> (11.45, 8.75)
  line L786 (11.45, 8.75) -> (11.3, 8.83) construction
  line L787 (11.3, 8.75) -> (11.45, 8.83) construction
  line L788 (11.45, 8.875) -> (11.3, 8.875)
  line L789 (11.3, 8.875) -> (11.3, 8.955)
  line L790 (11.3, 8.955) -> (11.45, 8.955)
  line L791 (11.45, 8.955) -> (11.45, 8.875)
  line L792 (11.45, 8.875) -> (11.3, 8.955) construction
  line L793 (11.3, 8.875) -> (11.45, 8.955) construction
  line L794 (11.45, 9) -> (11.3, 9)
  line L795 (11.3, 9) -> (11.3, 9.08)
  line L796 (11.3, 9.08) -> (11.45, 9.08)
  line L797 (11.45, 9.08) -> (11.45, 9)
  line L798 (11.45, 9) -> (11.3, 9.08) construction
  line L799 (11.3, 9) -> (11.45, 9.08) construction
  line L800 (11.45, 9.125) -> (11.3, 9.125)
  line L801 (11.3, 9.125) -> (11.3, 9.205)
  line L802 (11.3, 9.205) -> (11.45, 9.205)
  line L803 (11.45, 9.205) -> (11.45, 9.125)
  line L804 (11.45, 9.125) -> (11.3, 9.205) construction
  line L805 (11.3, 9.125) -> (11.45, 9.205) construction
  line L806 (11.45, 9.25) -> (11.3, 9.25)
  line L807 (11.3, 9.25) -> (11.3, 9.33)
  line L808 (11.3, 9.33) -> (11.45, 9.33)
  line L809 (11.45, 9.33) -> (11.45, 9.25)
  line L810 (11.45, 9.25) -> (11.3, 9.33) construction
  line L811 (11.3, 9.25) -> (11.45, 9.33) construction
  line L812 (11.45, 9.375) -> (11.3, 9.375)
  line L813 (11.3, 9.375) -> (11.3, 9.455)
  line L814 (11.3, 9.455) -> (11.45, 9.455)
  line L815 (11.45, 9.455) -> (11.45, 9.375)
  line L816 (11.45, 9.375) -> (11.3, 9.455) construction
  line L817 (11.3, 9.375) -> (11.45, 9.455) construction
  line L818 (11.45, 9.5) -> (11.3, 9.5)
  line L819 (11.3, 9.5) -> (11.3, 9.58)
  line L820 (11.3, 9.58) -> (11.45, 9.58)
  line L821 (11.45, 9.58) -> (11.45, 9.5)
  line L822 (11.45, 9.5) -> (11.3, 9.58) construction
  line L823 (11.3, 9.5) -> (11.45, 9.58) construction
  line L824 (11.45, 9.625) -> (11.3, 9.625)
  line L825 (11.3, 9.625) -> (11.3, 9.705)
  line L826 (11.3, 9.705) -> (11.45, 9.705)
  line L827 (11.45, 9.705) -> (11.45, 9.625)
  line L828 (11.45, 9.625) -> (11.3, 9.705) construction
  line L829 (11.3, 9.625) -> (11.45, 9.705) construction
  line L830 (11.45, 9.75) -> (11.3, 9.75)
  line L831 (11.3, 9.75) -> (11.3, 9.83)
  line L832 (11.3, 9.83) -> (11.45, 9.83)
  line L833 (11.45, 9.83) -> (11.45, 9.75)
  line L834 (11.45, 9.75) -> (11.3, 9.83) construction
  line L835 (11.3, 9.75) -> (11.45, 9.83) construction
  line L836 (11.5, 10.5) -> (-11.5, 10.5) projected
  line L837 (11.45, 9.875) -> (11.3, 9.875)
  line L838 (11.3, 9.875) -> (11.3, 9.955)
  line L839 (11.3, 9.955) -> (11.45, 9.955)
  line L840 (11.45, 9.955) -> (11.45, 9.875)
  line L841 (11.45, 9.875) -> (11.3, 9.955) construction
  line L842 (11.3, 9.875) -> (11.45, 9.955) construction
  line L843 (11.45, 10) -> (11.3, 10)
  line L844 (11.3, 10) -> (11.3, 10.08)
  line L845 (11.3, 10.08) -> (11.45, 10.08)
  line L846 (11.45, 10.08) -> (11.45, 10)
  line L847 (11.45, 10) -> (11.3, 10.08) construction
  line L848 (11.3, 10) -> (11.45, 10.08) construction
  line L849 (11.45, 10.125) -> (11.3, 10.125)
  line L850 (11.3, 10.125) -> (11.3, 10.205)
  line L851 (11.3, 10.205) -> (11.45, 10.205)
  line L852 (11.45, 10.205) -> (11.45, 10.125)
  line L853 (11.45, 10.125) -> (11.3, 10.205) construction
  line L854 (11.3, 10.125) -> (11.45, 10.205) construction
  point P0 (0, 0)
  point P1 (11.375, -7.46)
  point P2 (11.375, -7.335)
  point P3 (11.375, -7.21)
  point P4 (11.375, -7.085)
  point P5 (11.375, -6.96)
  point P6 (11.375, -6.835)
  point P7 (11.375, -6.71)
  point P8 (11.375, -6.585)
  point P9 (11.375, -6.46)
  point P10 (11.375, -6.335)
  point P11 (11.375, -6.21)
  point P12 (11.375, -6.085)
  point P13 (11.375, -5.96)
  point P14 (11.375, -5.835)
  point P15 (11.375, -5.71)
  point P16 (11.375, -5.585)
  point P17 (11.375, -5.46)
  point P18 (11.375, -5.335)
  point P19 (11.375, -5.21)
  point P20 (11.375, -5.085)
  point P21 (11.375, -4.96)
  point P22 (11.375, -4.835)
  point P23 (11.375, -4.71)
  point P24 (11.375, -4.585)
  point P25 (11.375, -4.46)
  point P26 (11.375, -4.335)
  point P27 (11.375, -4.21)
  point P28 (11.375, -4.085)
  point P29 (11.375, -3.96)
  point P30 (11.375, -3.835)
  point P31 (11.375, -3.71)
  point P32 (11.375, -3.585)
  point P33 (11.375, -3.46)
  point P34 (11.375, -3.335)
  point P35 (11.375, -3.21)
  point P36 (11.375, -3.085)
  point P37 (11.375, -2.96)
  point P38 (11.375, -2.835)
  point P39 (11.375, -2.71)
  point P40 (11.375, -2.585)
  point P41 (11.375, -2.46)
  point P42 (11.375, -2.335)
  point P43 (11.375, -2.21)
  point P44 (11.375, -2.085)
  point P45 (11.375, -1.96)
  point P46 (11.375, -1.835)
  point P47 (11.375, -1.71)
  point P48 (11.375, -1.585)
  point P49 (11.375, -1.46)
  point P50 (11.375, -1.335)
  point P51 (11.375, -1.21)
  point P52 (11.375, -1.085)
  point P53 (11.375, -0.96)
  point P54 (11.375, -0.835)
  point P55 (11.375, -0.71)
  point P56 (11.375, -0.585)
  point P57 (11.375, -0.46)
  point P58 (11.375, -0.335)
  point P59 (11.375, -0.21)
  point P60 (11.375, -0.085)
  point P61 (11.375, 0.04)
  point P62 (11.375, 0.165)
  point P63 (11.375, 0.29)
  point P64 (11.375, 0.415)
  point P65 (11.375, 0.54)
  point P66 (11.375, 0.665)
  point P67 (11.375, 0.79)
  point P68 (11.375, 0.915)
  point P69 (11.375, 1.04)
  point P70 (11.375, 1.165)
  point P71 (11.375, 1.29)
  point P72 (11.375, 1.415)
  point P73 (11.375, 1.54)
  point P74 (11.375, 1.665)
  point P75 (11.375, 1.79)
  point P76 (11.375, 1.915)
  point P77 (11.375, 2.04)
  point P78 (11.375, 2.165)
  point P79 (11.375, 2.29)
  point P80 (11.375, 2.415)
  point P81 (11.375, 2.54)
  point P82 (11.375, 2.665)
  point P83 (11.375, 2.79)
  point P84 (11.375, 2.915)
  point P85 (11.375, 3.04)
  point P86 (11.375, 3.165)
  point P87 (11.375, 3.29)
  point P88 (11.375, 3.415)
  point P89 (11.375, 3.54)
  point P90 (11.375, 3.665)
  point P91 (11.375, 3.79)
  point P92 (11.375, 3.915)
  point P93 (11.375, 4.04)
  point P94 (11.375, 4.165)
  point P95 (11.375, 4.29)
  point P96 (11.375, 4.415)
  point P97 (11.375, 4.54)
  point P98 (11.375, 4.665)
  point P99 (11.375, 4.79)
  point P100 (11.375, 4.915)
  point P101 (11.375, 5.04)
  point P102 (11.375, 5.165)
  point P103 (11.375, 5.29)
  point P104 (11.375, 5.415)
  point P105 (11.375, 5.54)
  point P106 (11.375, 5.665)
  point P107 (11.375, 5.79)
  point P108 (11.375, 5.915)
  point P109 (11.375, 6.04)
  point P110 (11.375, 6.165)
  point P111 (11.375, 6.29)
  point P112 (11.375, 6.415)
  point P113 (11.375, 6.54)
  point P114 (11.375, 6.665)
  point P115 (11.375, 6.79)
  point P116 (11.375, 6.915)
  point P117 (11.375, 7.04)
  point P118 (11.375, 7.165)
  point P119 (11.375, 7.29)
  point P120 (11.375, 7.415)
  point P121 (11.375, 7.54)
  point P122 (11.375, 7.665)
  point P123 (11.375, 7.79)
  point P124 (11.375, 7.915)
  point P125 (11.375, 8.04)
  point P126 (11.375, 8.165)
  point P127 (11.375, 8.29)
  point P128 (11.375, 8.415)
  point P129 (11.375, 8.54)
  point P130 (11.375, 8.665)
  point P131 (11.375, 8.79)
  point P132 (11.375, 8.915)
  point P133 (11.375, 9.04)
  point P134 (11.375, 9.165)
  point P135 (11.375, 9.29)
  point P136 (11.375, 9.415)
  point P137 (11.375, 9.54)
  point P138 (11.375, 9.665)
  point P139 (11.375, 9.79)
  point P140 (11.375, 9.915)
  point P141 (11.375, 10.04)
  point P142 (11.375, 10.165)
  dimension "d4" = 0.15
  dimension "d5" = 0.08
  dimension "d8" = 0.125
  dimension "d13" = 3
  dimension "d14" = 0.05
  dimension "d15" = 0.67
  constraints: 1704 end point, 284 midpoint, 2 parallel, 1 collinear, 1 horizontal, 1 perpendicular, 1 vertical, 1550 other
  measures "d4" distance of L3.end L4.end
  measures "d5" distance of L2.end L3.end
  measures "d8" distance of L2.start L8.start
  measures "d13" distance between parallel lines of L1 L2
  measures "d14" distance between parallel lines of L5 L0
  measures "d15" distance between parallel lines of L832 L836
extrude "Extrusion2" add sketch "Sketch3" along normal blind 0.01
body "Solid1"
